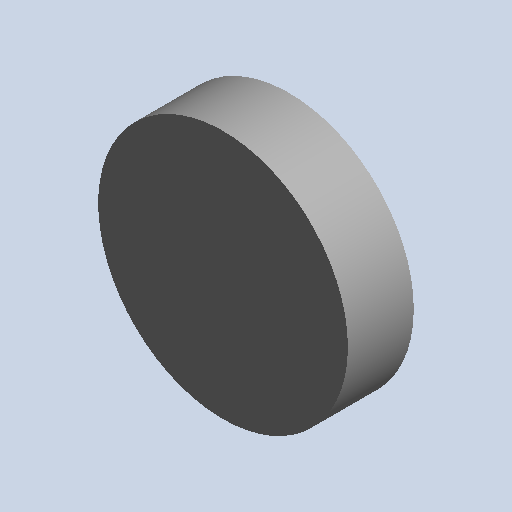
# Autodesk Inventor part: LIdar_p1
Saved by Autodesk Inventor 2026 (Build 300175050, 175E)
## iProperties
Part Number: LIdar_p1
Material: Generic
Document SubType Name: Modeling
Designer: Kartik
Mass: 77.3586 g
Surface Area: 124.407 cm^2
Volume: 77.3586 cm^3
Density: 1 g/cm^3
Appearance: Default
Author: Kartik
Autodesk Inventor part; units mm, degrees
ref_plane "YZ Plane" through (0, 0, 0) normal (1, 0, 0) x (0, 1, 0)
ref_plane "XZ Plane" through (0, 0, 0) normal (0, 1, 0) x (-1, 0, 0)
ref_plane "XY Plane" through (0, 0, 0) normal (0, 0, 1) x (1, 0, 0)
sketch "Sketch1" plane through (0, 0, 0) normal (0, 0, 1) x (1, 0, 0)
  circle A0 centre (0, 0) radius 36
  dimension "d0" = 72
  constraints: 1 centre point, 1 coincident
  measures "d0" diameter of A0
extrude "Extrusion1" add sketch "Sketch1" along normal blind 19
body "Solid1"
